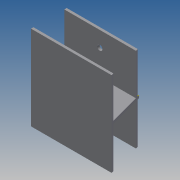
# Autodesk Inventor part: endChannel
Saved by Autodesk Inventor 2014 SP1 (Build 180222100, 222)
## iProperties
Created: 2014-05-20
Part Number: endChannel
Material: Generic
Document SubType Name: Modeling
Designer: Dave
Density: 1 g/cm^3
Appearance: Default
Author: Dave
Autodesk Inventor part; units mm, degrees
ref_plane "YZ Plane" through (0, 0, 0) normal (1, 0, 0) x (0, 1, 0)
ref_plane "XZ Plane" through (0, 0, 0) normal (0, 1, 0) x (-1, 0, 0)
ref_plane "XY Plane" through (0, 0, 0) normal (0, 0, 1) x (1, 0, 0)
sketch "Sketch2" plane through (0, 0, 0) normal (1, 0, 0) x (0, 1, 0)
  line L0 (0, 0) -> (0, 12.7) construction
  line L1 (-1.524, 0) -> (1.524, 0) construction
  line L2 (-1.524, 0) -> (-52.324, 0)
  line L3 (-52.324, 0) -> (-52.324, -3.048)
  line L4 (-52.324, -3.048) -> (52.324, -3.048)
  line L5 (52.324, -3.048) -> (52.324, 0)
  line L6 (52.324, 0) -> (1.524, 0)
  line L7 (0, 19.05) -> (17.4058, 19.05) construction
  line L8 (-1.524, 38.1) -> (-52.324, 38.1)
  line L9 (-52.324, 38.1) -> (-52.324, 41.148)
  line L10 (-52.324, 41.148) -> (52.324, 41.148)
  line L11 (52.324, 41.148) -> (52.324, 38.1)
  line L12 (52.324, 38.1) -> (1.524, 38.1)
  line L13 (-1.524, 38.1) -> (-1.524, 0)
  line L14 (1.524, 38.1) -> (1.524, 0)
  dimension "d2" = 12.7
  dimension "d3" = 3.048
  dimension "d4" = 50.8
  dimension "d5" = 3.048
  dimension "d6" = 104.648
  dimension "d7" = 90
  dimension "d9" = 19.05
  constraints: 30 end point, 6 parallel, 6 symmetric about line, 2 perpendicular, 1 collinear, 1 midpoint, 1 vertical
  measures "d2" distance of L0.start L0.end
  measures "d3" distance of L1.start L1.end
  measures "d4" distance of L1.start L2.end
  measures "d5" distance of L2.end L3.end
  measures "d6" distance of L3.end L4.end
  measures "d7" angle of L4 L3
  measures "d9" distance between parallel lines of L6 L7
extrude "Extrusion1" add sketch "Sketch2" along normal blind 101.6
ref_plane "Work Plane1" through (101.6, -52.324, -3.048) normal (0.9659258, 0, -0.258819) x (0, 1, 0)
sketch "Sketch3" plane through (101.6, -52.324, -3.048) normal (0.9659258, 0, -0.258819) x (0, 1, 0)
  line L0 (-5.9321, -28.1882) -> (161.3801, -28.1882)
  line L1 (161.3801, -28.1882) -> (161.3801, 44.7495)
  line L2 (161.3801, 44.7495) -> (-5.9321, 44.7495)
  line L3 (-5.9321, 44.7495) -> (-5.9321, -28.1882)
  point P0 (52.324, -23.3519)
  constraints: 8 end point, 2 parallel, 1 horizontal, 1 perpendicular
extrude "Extrusion2" cut sketch "Sketch3" against normal blind 13.208
sketch "Sketch4" plane through (0, 1.524, 38.1) normal (0, 1, 0) x (1, 0, 0)
  line L0 (0, 38.1) -> (0, 0) projected
  line L1 (76.2, 9.525) -> (79.248, 9.525)
  line L2 (79.248, 9.525) -> (79.248, 28.575)
  line L3 (79.248, 28.575) -> (76.2, 28.575)
  line L4 (76.2, 28.575) -> (76.2, 9.525)
  line L5 (0, 19.05) -> (76.2, 19.05) construction
  dimension "d15" = 3.048
  dimension "d16" = 19.05
  dimension "d17" = 76.2
  constraints: 10 end point, 2 midpoint, 2 parallel, 2 perpendicular, 1 horizontal
  measures "d15" distance of L3.end L2.end
  measures "d16" distance of L2.end L1.end
  measures "d17" distance of L5.end L5.start
extrude "Extrusion3" [suppressed]
sketch "Sketch5" plane through (0, 1.524, 38.1) normal (0, 1, 0) x (1, 0, 0)
  line L0 (76.2, 9.525) -> (50.8, 9.525)
  line L1 (50.8, 9.525) -> (50.8, 28.575)
  line L2 (50.8, 28.575) -> (76.2, 28.575)
  line L3 (76.2, 28.575) -> (76.2, 9.525)
  dimension "d20" = 25.4
  constraints: 8 end point, 2 parallel, 1 horizontal, 1 perpendicular
  measures "d20" distance of L1.end L2.end
extrude "Extrusion4" [suppressed]
sketch "Sketch6" plane through (0, -52.324, -3.048) normal (0, 0, -1) x (-1, 0, 0)
  line L0 (0, 0) -> (-87.9261, 0) projected
  line L1 (0, 104.648) -> (-87.9261, 104.648) projected
  circle A0 centre (-43.963, 85.598) radius 3.175
  circle A1 centre (-43.963, 19.05) radius 3.175
  point P0 (0, 52.324)
  dimension "d23" = 6.35
  dimension "d24" = 6.35
  dimension "d25" = 19.05
  dimension "d26" = 19.05
  constraints: 2 centre point
  measures "d23" diameter of A0
  measures "d24" diameter of A1
  measures "d25" distance from line of A0.centre L1
  measures "d26" distance from line of A1.centre L0
hole "Hole1" at (43.963, 33.274, -3.048) at (43.963, -33.274, -3.048) direction (0, 0, 1) diameter 6.35 depth 25.4 tip angle 118
ref_plane "Work Plane2" through (88.8421, -52.324, 0.3705) normal (0.9659258, 0, -0.258819) x (0, 1, 0)
sketch "Sketch7" plane through (88.8421, -52.324, 0.3705) normal (0.9659258, 0, -0.258819) x (0, 1, 0)
  line L0 (50.8, -5.588) -> (53.848, -5.588)
  line L1 (53.848, -5.588) -> (53.848, -3.048)
  line L2 (53.848, -3.048) -> (50.8, -3.048)
  line L3 (50.8, -3.048) -> (50.8, -5.588)
  line L4 (50.8, -0.3836) -> (50.8, 39.0605) projected
  point P0 (52.324, -23.3519)
  dimension "d35" = 3.048
  dimension "d36" = 2.54
  dimension "d39" = 0
  constraints: 8 end point, 2 parallel, 1 horizontal, 1 perpendicular
  measures "d35" distance of L2.end L1.end
  measures "d36" distance of L1.end L0.end
  measures "d39" distance between parallel lines of L4 L3
extrude "DRAWING_ONLY_ALIGN" add sketch "Sketch7" against normal blind 7.62
body "Solid1"
